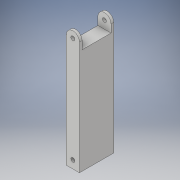
# Autodesk Inventor part: brazo 1
Saved by Autodesk Inventor 2019 (Build 230136000, 136)
## iProperties
Created: 2019-10-18
Part Number: brazo 1
Material: Genérico
Document SubType Name: Modeling
Designer: Josue
Density: 1 g/cm^3
Appearance: Valor por defecto
Author: Josue
Autodesk Inventor part; units mm, degrees
ref_plane "YZ Plane" through (0, 0, 0) normal (1, 0, 0) x (0, 1, 0)
ref_plane "XZ Plane" through (0, 0, 0) normal (0, 1, 0) x (-1, 0, 0)
ref_plane "XY Plane" through (0, 0, 0) normal (0, 0, 1) x (1, 0, 0)
sketch "Boceto1" plane through (0, 0, 0) normal (0, 1, 0) x (-1, 0, 0)
  line L0 (-25, 65) -> (25, 65)
  line L1 (25, 65) -> (25, -65)
  line L2 (25, -65) -> (-25, -65)
  line L3 (-25, -65) -> (-25, 65)
  line L4 (-25, 65) -> (25, -65) construction
  line L5 (25, 65) -> (-25, -65) construction
  point P0 (0, 0)
  dimension "d0" = 50
  dimension "d1" = 130
  constraints: 12 end point, 2 midpoint, 2 parallel, 1 horizontal, 1 perpendicular
  measures "d0" distance of L1.end L2.end
  measures "d1" distance of L0.end L1.end
extrude "Extrusión1" add sketch "Boceto1" along normal blind 400
sketch "Boceto2" plane through (-25, 0, 65) normal (0, 0, 1) x (1, 0, 0)
  line L0 (0, 400) -> (50, 400) projected
  line L1 (0, 400) -> (0, 430)
  line L2 (50, 400) -> (50, 430)
  arc A0 (50, 430) -> (0, 430) centre (25, 430) ccw
  circle A1 centre (25, 430) radius 7.5
  point P0 (25, 0)
  dimension "d4" = 30
  dimension "d5" = 30
  dimension "d6" = 15
  constraints: 4 end point, 2 centre point, 2 point on circle, 2 vertical, 1 coincident, 1 tangent
  measures "d4" distance of L0.start L1.end
  measures "d5" distance of L0.end L2.end
  measures "d6" diameter of A1
extrude "Extrusión2" add sketch "Boceto2" against normal blind 10
sketch "Boceto3" plane through (25, 0, -65) normal (0, 0, -1) x (-1, 0, 0)
  arc A0 (50, 430) -> (0, 430) centre (25, 430) ccw projected
  circle A1 centre (25, 430) radius 7.5 projected
  line L0 (50, 400) -> (50, 430) projected
  line L1 (0, 400) -> (50, 400) projected
  line L2 (0, 430) -> (0, 400) projected
  point P0 (25, 0)
extrude "Extrusión3" add sketch "Boceto3" against normal blind 10
sketch "Boceto4" plane through (25, 0, -65) normal (0, 0, -1) x (-1, 0, 0)
  line L0 (25, 0) -> (25, 30)
  circle A0 centre (25, 30) radius 7.5
  dimension "d11" = 30
  dimension "d12" = 15
  constraints: 2 end point, 1 centre point, 1 coincident, 1 vertical
  measures "d11" distance of L0.start L0.end
  measures "d12" diameter of A0
extrude "Extrusión4" cut sketch "Boceto4" against normal up to next
